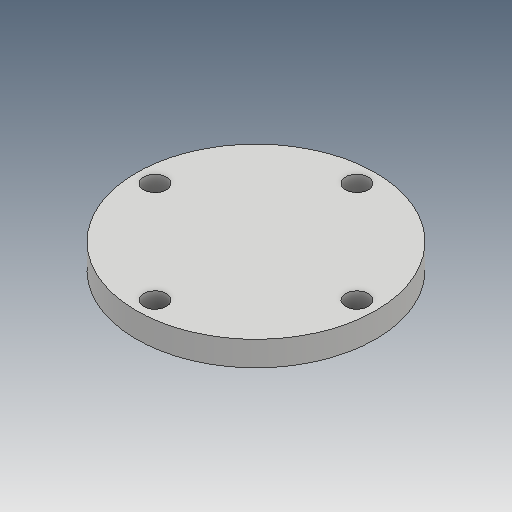
# Autodesk Inventor part: 접촉부 철판가공
Saved by Autodesk Inventor 2018 (Build 220112000, 112)
## iProperties
Created: 2018-10-26
Part Number: 접촉부 철판가공
Material: 일반
Document SubType Name: Modeling
Designer: dhksr
Density: 1 g/cm^3
Appearance: 기본값
Author: dhksr
Autodesk Inventor part; units mm, degrees
ref_plane "YZ Plane" through (0, 0, 0) normal (1, 0, 0) x (0, 1, 0)
ref_plane "XZ Plane" through (0, 0, 0) normal (0, 1, 0) x (-1, 0, 0)
ref_plane "XY Plane" through (0, 0, 0) normal (0, 0, 1) x (1, 0, 0)
sketch "스케치1" plane through (0, 0, 0) normal (0, 0, 1) x (1, 0, 0)
  circle A0 centre (0, 0) radius 29
  circle A1 centre (-24.5, 0) radius 1.5
  circle A2 centre (-24.5, 0) radius 2.75
  circle A3 centre (0, -24.5) radius 1.5
  circle A4 centre (0, -24.5) radius 2.75
  circle A5 centre (24.5, 0) radius 1.5
  circle A6 centre (24.5, 0) radius 2.75
  circle A7 centre (0, 24.5) radius 1.5
  circle A8 centre (0, 24.5) radius 2.75
  dimension "d0" = 58
  dimension "d1" = 3
  dimension "d2" = 5.5
  dimension "d3" = 24.5
  dimension "d6" = 360
  constraints: 9 centre point, 5 coincident, 17 other
  measures "d0" diameter of A0
  measures "d1" diameter of A1
  measures "d2" diameter of A2
  measures "d3" distance of point (0, 0) A1.centre
extrude "돌출1" add sketch "스케치1" along normal blind 6 contours A0 | A2 | A4 | A6 | A8
sketch "스케치2" plane through (0, 0, 6) normal (0, 0, 1) x (1, 0, 0)
  circle A0 centre (0, 24.5) radius 1.5 projected
  circle A1 centre (24.5, 0) radius 1.5 projected
  circle A2 centre (0, -24.5) radius 1.5 projected
  circle A3 centre (-24.5, 0) radius 1.5 projected
  circle A4 centre (-24.5, 0) radius 2.75 projected
  circle A5 centre (24.5, 0) radius 2.75 projected
  circle A6 centre (0, -24.5) radius 2.75 projected
  circle A7 centre (0, 24.5) radius 2.75 projected
extrude "돌출2" cut sketch "스케치2" against normal blind 4
sketch "스케치5" plane through (0, 0, 0) normal (0, 0, -1) x (-1, 0, 0)
  circle A0 centre (0, 0) radius 65 projected
  circle A1 centre (7.157, 23.4313) radius 1 projected
  line L0 (22.2881, 36.3872) -> (18.0584, 32.156) projected
  arc A2 (18.0584, 32.156) -> (18.0588, 29.3276) centre (19.4728, 30.742) ccw projected
  line L1 (18.0588, 29.3276) -> (29.3745, 18.0158) projected
  arc A3 (29.3745, 18.0158) -> (32.2029, 18.0163) centre (30.7884, 19.4302) ccw projected
  line L2 (32.2029, 18.0163) -> (36.4326, 22.2474) projected
  arc A4 (36.4326, 22.2474) -> (36.4322, 25.0758) centre (35.0182, 23.6614) ccw projected
  line L3 (36.4322, 25.0758) -> (25.1165, 36.3876) projected
  arc A5 (25.1165, 36.3876) -> (22.2881, 36.3872) centre (23.7025, 34.9732) ccw projected
  circle A6 centre (0, 24.5) radius 1.2295 projected
  circle A7 centre (-24.5, 0) radius 1.2295 projected
  circle A8 centre (0, -24.5) radius 1.2295 projected
  circle A9 centre (24.5, 0) radius 1.2295 projected
  circle A10 centre (0, 51.0531) radius 2.5 projected
  circle A11 centre (0, -51.0531) radius 2.5 projected
  circle A12 centre (-51.0531, 0) radius 2.5 projected
  circle A13 centre (51.0531, 0) radius 2.5 projected
  circle A14 centre (-22.9994, -55.4169) radius 1.5 projected
  circle A15 centre (55.4169, -22.9994) radius 1.5 projected
  circle A16 centre (22.9994, 55.4169) radius 1.5 projected
  circle A17 centre (-55.4169, 22.9994) radius 1.5 projected
  circle A18 centre (-22.9226, 55.4487) radius 1.5 projected
  circle A19 centre (55.4487, 22.9226) radius 1.5 projected
  circle A20 centre (22.9226, -55.4487) radius 1.5 projected
  circle A21 centre (-55.4487, -22.9226) radius 1.5 projected
  circle A22 centre (0, 0) radius 65 projected
  circle A23 centre (0, 0) radius 25
  line L4 (-20.0138, -19.9861) -> (19.9861, -20.0138) projected
  line L5 (19.9861, -20.0138) -> (20.0138, 19.9861) projected
  line L6 (20.0138, 19.9861) -> (-19.9861, 20.0138) projected
  line L7 (-19.9861, 20.0138) -> (-20.0138, -19.9861) projected
  circle A24 centre (24.3126, 5.8222) radius 1
  dimension "d14" = 50
  dimension "d15" = 2
  constraints: 1 centre point, 1 coincident, 3 other
  measures "d15" diameter of A24
extrude "돌출3" cut sketch "스케치5" against normal blind 3 contours A24 A23 | A23 A24
